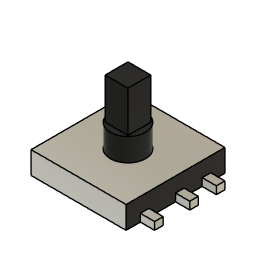
5way_SMD_Switch (Autodesk Fusion 360 design; units mm, degrees)
Autodesk Fusion 360 part; units mm, degrees
sketch "Sketch1" plane through (0, 0, 0) normal (0, 0, 1) x (1, 0, 0)
  line L0 (5, -5.2) -> (-5, -5.2)
  line L1 (-5, -5.2) -> (-5, 5.2)
  line L2 (-5, 5.2) -> (5, 5.2)
  line L3 (5, 5.2) -> (5, -5.2)
  line L4 (5, -5.2) -> (-5, 5.2) construction
  line L5 (-5, -5.2) -> (5, 5.2) construction
  line L6 (0, 0) -> (6.5, 0) construction
  line L7 (6.5, 0) -> (6.5, 5.2) construction
  line L8 (6.5, 0) -> (5, 0)
  line L9 (5, 0) -> (5, 0.9)
  line L10 (5, 0.9) -> (6.5, 0.9)
  line L11 (6.5, 0.9) -> (6.5, 0)
  line L12 (6.5, 0.45) -> (6.5, 3.25) construction
  line L13 (6.5, 3.25) -> (5, 3.25) construction
  line L14 (6.5, 2.8) -> (5, 2.8)
  line L15 (5, 2.8) -> (5, 3.7)
  line L16 (5, 3.7) -> (6.5, 3.7)
  line L17 (6.5, 3.7) -> (6.5, 2.8)
  line L18 (6.5, 2.8) -> (5, 3.7) construction
  line L19 (5, 2.8) -> (6.5, 3.7) construction
  line L20 (6.5, 0.45) -> (6.5, -3.25) construction
  line L21 (6.5, -3.25) -> (5, -3.25) construction
  line L22 (6.5, -2.8) -> (5, -2.8)
  line L23 (5, -2.8) -> (5, -3.7)
  line L24 (5, -3.7) -> (6.5, -3.7)
  line L25 (6.5, -3.7) -> (6.5, -2.8)
  line L26 (6.5, -2.8) -> (5, -3.7) construction
  line L27 (5, -2.8) -> (6.5, -3.7) construction
  line L28 (0, 2.5) -> (0, 20)
  line L29 (-5, 2.8) -> (-5, 3.7)
  line L30 (-6.5, 0.9) -> (-6.5, 0)
  line L31 (-6.5, -3.25) -> (-5, -3.25) construction
  line L32 (-6.5, -2.8) -> (-5, -3.7) construction
  line L33 (-6.5, 3.25) -> (-5, 3.25) construction
  line L34 (-6.5, 0) -> (-5, 0)
  line L35 (-6.5, 3.7) -> (-6.5, 2.8)
  line L36 (-5, -2.8) -> (-5, -3.7)
  line L37 (-5, -2.8) -> (-6.5, -3.7) construction
  line L38 (-6.5, -2.8) -> (-5, -2.8)
  line L39 (-6.5, 0.45) -> (-6.5, -3.25) construction
  line L40 (-5, 2.8) -> (-6.5, 3.7) construction
  line L41 (-6.5, 0.45) -> (-6.5, 3.25) construction
  line L42 (-5, 3.7) -> (-6.5, 3.7)
  line L43 (-5, 0.9) -> (-6.5, 0.9)
  line L44 (-6.5, 2.8) -> (-5, 2.8)
  line L45 (-5, 0) -> (-5, 0.9)
  line L46 (-6.5, -3.7) -> (-6.5, -2.8)
  line L47 (-5, -3.7) -> (-6.5, -3.7)
  line L48 (-6.5, 2.8) -> (-5, 3.7) construction
  point P0 (5.75, 3.25)
  point P1 (5.75, -3.25)
  point P2 (-5.75, -3.25)
  point P3 (-5.75, 3.25)
  dimension "d1" = 10
  dimension "d2" = 10.4
  dimension "d3" = 6.5
  dimension "d4" = 0.9
  dimension "d5" = 2.8
  dimension "d6" = 0.9
  dimension "d7" = 3.7
  dimension "d8" = 0.9
  constraint horizontal L0
  constraint perpendicular L0 L1
  constraint parallel L0 L2
  constraint parallel L1 L3
  constraint coincident L4 L6.start
  constraint coincident L5 L6.start
  constraint coincident L6.start origin
  constraint perpendicular L3 L6
  constraint perpendicular L2 L7
  constraint horizontal L8
  constraint vertical L9
  constraint horizontal L10
  constraint vertical L11
  constraint coincident L3 L9.end
  constraint midpoint L11 L12.start
  constraint perpendicular L10 L12
  constraint perpendicular L7 L13
  constraint horizontal L14
  constraint perpendicular L14 L15
  constraint parallel L14 L16
  constraint parallel L15 L17
  constraint coincident L18 P0
  constraint coincident L19 P0
  constraint midpoint L13 P0
  constraint perpendicular L8 L20
  constraint coincident L3 L21.end
  constraint perpendicular L3 L21
  constraint horizontal L22
  constraint perpendicular L22 L23
  constraint parallel L22 L24
  constraint parallel L23 L25
  constraint coincident L26 P1
  constraint coincident L27 P1
  constraint coincident L20 L22.start
  constraint midpoint L21 P1
  constraint symmetric L6.end L28 L30.end
  constraint symmetric L8.end L28 L34.end
  constraint symmetric L9.end L28 L43.start
  constraint symmetric L10.end L28 L30.start
  constraint symmetric L12.start L28 L39.start
  constraint symmetric L12.end L28 L33.start
  constraint symmetric L13.end L28 L33.end
  constraint symmetric L14.start L28 L35.end
  constraint symmetric L14.end L28 L29.start
  constraint symmetric L15.end L28 L29.end
  constraint symmetric L16.end L28 L35.start
  constraint symmetric P0 L28 P3
  constraint symmetric L20.end L28 L31.start
  constraint symmetric L21.end L28 L31.end
  constraint symmetric L22.start L28 L32.start
  constraint symmetric L22.end L28 L36.start
  constraint symmetric L23.end L28 L32.end
  constraint symmetric L24.end L28 L37.end
  constraint symmetric P1 L28 P2
  measures "d1" distance of L1.end L2.end
  measures "d2" distance of L0.end L1.end
  measures "d3" distance of L6.start L6.end
  measures "d4" distance of L6.end L10.end
  measures "d5" distance of L12.start L12.end
  measures "d6" distance of L14.end L15.end
  measures "d7" distance of L12.start L20.end
  measures "d8" distance of L22.end L23.end
extrude "Extrude1" add sketch "Sketch1" along normal blind 2.35 contours L0 L1 L2 L3 L9 L15 L23 L29 L36 L45 makes body 1
extrude "Extrude2" add sketch "Sketch1" along normal blind 0.8 separate body contours L3 L22 L23 L24 L25 | L1 L36 L38 L46 L47 | L3 L8 L9 L10 L11 | L1 L30 L34 L43 L45 | L3 L14 L15 L16 L17 | L1 L29 L35 L42 L44 makes body 2 at (-5.5, 3.1, 0) makes body 3 at (6, 3.4, 0) makes body 4 at (-5.5, 0.3, 0) makes body 5 at (5.5, -3.1, 0) makes body 6 at (5.5, 0.6, 0) makes body 7 at (-6, -3.4, 0)
sketch "Sketch2" plane through (0, 0, 2.35) normal (0, 0, 1) x (-1, 0, 0)
  line L0 (5, -5.2) -> (5, 5.2)
  line L1 (5, 5.2) -> (-5, 5.2)
  line L2 (-5, 5.2) -> (-5, -5.2)
  line L3 (-5, -5.2) -> (5, -5.2)
  circle A0 centre (0, 0) radius 1.85
  line L4 (-1.2, 1.2) -> (1.2, 1.2)
  line L5 (1.2, 1.2) -> (1.2, -1.2)
  line L6 (1.2, -1.2) -> (-1.2, -1.2)
  line L7 (-1.2, -1.2) -> (-1.2, 1.2)
  line L8 (-1.2, 1.2) -> (1.2, -1.2) construction
  line L9 (1.2, 1.2) -> (-1.2, -1.2) construction
  dimension "d13" = 3.7
  dimension "d14" = 2.4
  dimension "d15" = 2.4
  constraint coincident A0.centre origin
  constraint horizontal L4
  constraint perpendicular L4 L5
  constraint parallel L4 L6
  constraint parallel L5 L7
  constraint coincident L8 A0.centre
  constraint coincident L9 A0.centre
  measures "d13" diameter of A0
  measures "d14" distance of L5.end L6.end
  measures "d15" distance of L4.end L5.end
extrude "Extrude3" add sketch "Sketch2" along normal blind 6.7 contours L4 L5 L6 L7 bodies 1
extrude "Extrude4" add sketch "Sketch2" along normal blind 2.4 contours A0 bodies 1
sketch "Sketch3" plane through (0, 0, 0) normal (0, 0, -1) x (1, 0, 0)
  line L0 (-5, 5.2) -> (-5, -5.2)
  line L1 (-5, -5.2) -> (5, -5.2)
  line L2 (5, -5.2) -> (5, 5.2)
  line L3 (5, 5.2) -> (-5, 5.2)
  line L4 (-1.2, -1.2) -> (-1.2, 1.2) construction
  line L5 (0, 0) -> (-2.2, 0) construction
  line L6 (-2.2, 0) -> (-2.2, -2.2) construction
  line L7 (-2.2, -2.2) -> (2.2, -2.2) construction
  circle A0 centre (2.2, -2.2) radius 0.35
  circle A1 centre (-2.2, -2.2) radius 0.35
  dimension "d20" = 2.2
  dimension "d21" = 2.2
  dimension "d22" = 4.4
  dimension "d23" = 0.7
  dimension "d24" = 0.7
  constraint coincident L5.start origin
  constraint perpendicular L4 L5
  constraint perpendicular L5 L6
  constraint perpendicular L6 L7
  constraint coincident L7.end A0.centre
  constraint coincident L6.end L7.start
  measures "d20" distance of L5.start L5.end
  measures "d21" distance of L5.end L6.end
  measures "d22" distance of L6.end L7.end
  measures "d23" diameter of A0
  measures "d24" diameter of A1
extrude "Extrude5" add sketch "Sketch3" along normal blind 0.6 contours A0 | A1 bodies 1
